Autodesk Fusion 360 part; units mm, degrees
(part 2 of 2)
sketch "Sketch1 (2)" plane through (0, 0, -40.7) normal (0, 0, -1) x (1, 0, 0) in component "Foot"
  circle A0 centre (-60, -22.7388) radius 1.25
  circle A1 centre (60, -2.7388) radius 1.25
  circle A2 centre (-60, -2.7388) radius 1.25
  circle A3 centre (60, -22.7388) radius 1.25
  arc A4 (100.5972, -6.0544) -> (100.9, -4.1886) centre (95, -4.1886) ccw
  line L0 (100.9, -4.1886) -> (100.9, 60)
  arc A5 (100.9, 60) -> (95, 65.9) centre (95, 60) ccw
  line L1 (95, 65.9) -> (-95, 65.9)
  arc A6 (-95, 65.9) -> (-100.9, 60) centre (-95, 60) ccw
  line L2 (-100.9, 60) -> (-100.9, -4.1886)
  arc A7 (-100.9, -4.1886) -> (-100.5972, -6.0544) centre (-95, -4.1886) ccw
  line L3 (-100.5972, -6.0544) -> (-91.9934, -31.8657)
  arc A8 (-91.9934, -31.8657) -> (-86.3962, -35.9) centre (-86.3962, -30) ccw
  line L4 (-86.3962, -35.9) -> (86.3962, -35.9)
  arc A9 (86.3962, -35.9) -> (91.9934, -31.8657) centre (86.3962, -30) ccw
  line L5 (91.9934, -31.8657) -> (100.5972, -6.0544)
  circle A10 centre (-60, -2.7388) radius 1.6
  circle A11 centre (-60, -22.7388) radius 1.6
  line L6 (-60, -2.7388) -> (-60, -22.7388) construction
  line L7 (-48, 1.2612) -> (-72, 1.2612)
  line L8 (-72, 1.2612) -> (-72, -26.7388)
  line L9 (-72, -26.7388) -> (-48, -26.7388)
  line L10 (-48, -26.7388) -> (-48, 1.2612)
  line L11 (-48, 1.2612) -> (-72, -26.7388) construction
  line L12 (-72, 1.2612) -> (-48, -26.7388) construction
  line L13 (-48, -18.7388) -> (-72, -18.7388)
  line L14 (-72, -18.7388) -> (-72, -6.7388)
  line L15 (-72, -6.7388) -> (-48, -6.7388)
  line L16 (-48, -6.7388) -> (-48, -18.7388)
  line L17 (-48, -18.7388) -> (-72, -6.7388) construction
  line L18 (-72, -18.7388) -> (-48, -6.7388) construction
  point P0 (-60, -12.7388)
  point P1 (-60, -12.7388)
  point P2 (-60, -12.7388)
  dimension "d1885" = 3.2
  dimension "d1886" = 3.2
  dimension "d1887" = 20
  dimension "d1888" = 24
  dimension "d1889" = 28
  dimension "d1890" = 24
  dimension "d1891" = 12
  constraint concentric A2 A10
  constraint concentric A0 A11
  constraint coincident A2.centre A10.centre
  constraint coincident A0.centre A11.centre
  constraint midpoint L6 P2
  constraint horizontal L7
  constraint perpendicular L7 L8
  constraint parallel L7 L9
  constraint parallel L8 L10
  constraint coincident L11 P2
  constraint coincident L12 P2
  constraint coincident P2 P1
  constraint horizontal L13
  constraint perpendicular L13 L14
  constraint parallel L13 L15
  constraint parallel L14 L16
  constraint coincident L17 P2
  constraint coincident L18 P2
  measures "d1885" diameter of A10
  measures "d1886" diameter of A11
  measures "d1887" distance of A2.centre A0.centre
  measures "d1888" distance of L8.end L9.end
  measures "d1889" distance of L7.end L8.end
  measures "d1890" distance of L14.end L15.end
  measures "d1891" distance of L13.end L14.end
extrude "Extrude1''" add sketch "Sketch1 (2)" along normal blind 50 separate body contours L8 L10 L13 L14 L15 L16 makes body 5 in component "Foot"
extrude "Extrude2''" add sketch "Sketch1 (2)" along normal blind 2.7 contours L7 L8 L10 L15 | L8 L10 L13 L14 L15 L16 | L8 L9 L10 L13 bodies 5 in component "Foot"
fillet "Fillet1" radius 6 2 edges at (-60, 6.7388, -90.7) (-60, 18.7388, -90.7) on bodies 5 in component "Foot"
chamfer "Chamfer1''" distance 10 distance2 5 1 edges at (-60, 18.7388, -43.4) measured on face at (-56, 18.7388, -57.1671) on bodies 5 in component "Foot"
chamfer "Chamfer2'" distance 10 distance2 5 1 edges at (-60, 6.7388, -43.4) measured on face at (-64, 6.7388, -57.1671) on bodies 5 in component "Foot"
sketch "Sketch2 (2)" plane through (0, 0, -43.4) normal (0, 0, -1) x (1, 0, 0) in component "Foot"
  line L0 (-48, -1.7388) -> (-48, 1.2612)
  line L1 (-48, 1.2612) -> (-72, 1.2612)
  line L2 (-72, 1.2612) -> (-72, -1.7388)
  circle A0 centre (-60, -2.7388) radius 3
  circle A1 centre (-60, -22.7388) radius 3
  line L3 (-72, -1.7388) -> (-61.249, -1.7388)
  arc A2 (-58.751, -1.7388) -> (-61.249, -1.7388) centre (-60, -2.7388) ccw
  line L4 (-58.751, -1.7388) -> (-48, -1.7388)
  dimension "d1899" = 6
  dimension "d1900" = 6
  dimension "d1901" = 20
  measures "d1899" diameter of A0
  measures "d1900" diameter of A1
  measures "d1901" distance of A0.centre A1.centre
extrude "Extrude3'" cut sketch "Sketch2 (2)" along normal blind 15 contours A0 L3 A2 L4 | A0 L3 A2 L4 | A1 bodies 5 in component "Foot"
fillet "Fillet2'" radius 1.2 19 edges at (-48, 21.2388, -48.4) (-48, 18.7388, -69.05) (-48, 12.7388, -90.7) (-48, 6.7388, -69.05) (-48, 4.2388, -48.4) (-48, 0.2388, -43.4) (-48, 26.7388, -42.05) (-60, 26.7388, -43.4) (-48, 25.2388, -43.4) (-48, -1.2612, -42.05) (-72, 6.7388, -69.05) (-72, 12.7388, -90.7) (-72, 18.7388, -69.05) (-72, 4.2388, -48.4) (-72, 0.2388, -43.4) (-60, -1.2612, -43.4) (-72, 26.7388, -42.05) (-72, 25.2388, -43.4) (-72, 21.2388, -48.4) on bodies 5 in component "Foot"
extrude "Extrude9'" cut sketch "Sketch2" against normal blind 1.35 contours L18 L19 L20 L21 bodies 2 in component "Cover (2)"
component "Case" placed x (1, 0, 0) y (0, 1, 0) z (0, 0, 1) at (0, 0, 0)
component "Cover (2)" placed x (1, 0, 0) y (0, 1, 0) z (0, 0, 1) at (0, 0, 0)
component "Foot" placed x (1, 0, 0) y (0, 1, 0) z (0, 0, 1) at (0, 0, 0)
equation "d1592 = lcd_display_width"
equation "d1679 = -remote_height"
equation "d1681 = remote_shell"
equation "d1713 = remote_shell * 2"
equation "d1728 = remote_shell * 2"
equation "d1730 = remote_shell * 2"
equation "d1750 = remote_shell"
equation "d1754 = remote_shell * 2"
equation "d1767 = remote_shell"
equation "d1771 = remote_shell * 2 / 3"
equation "d1779 = remote_shell * 2 / 3"
equation "d1793 = -remote_shell - remote_gap"
equation "d1800 = remote_shell * 2 / 3"
equation "d1804 = ( 35 / 2 ) * 1 mm"
equation "d1811 = 11 mm - 0.8 mm"
equation "d1812 = 7.5 mm - 1.2 mm"
equation "d1841 = remote_shell"
equation "d1852 = remote_shell"
equation "d1866 = -( 4.5 mm - remote_shell )"
equation "d1883 = -remote_shell - 5.00 mm"
equation "d1894 = remote_shell"
equation "d1911 = -remote_shell / 2"
equation "d1913 = remote_shell + remote_gap"
equation "lcd_display_width = 80 mm"
equation "remote_shell = 2.7 mm"
equation "remote_gap = 0.2 mm"
equation "remote_height = 38 mm"
named bodies: "Case", "Lid", "Foot"
